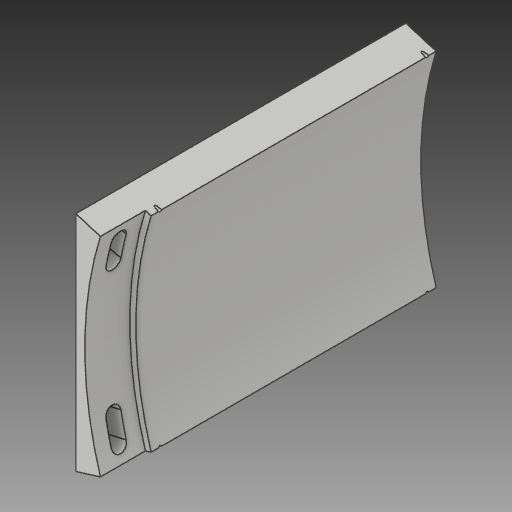
# Autodesk Inventor part: accesorios separador 1
Saved by Autodesk Inventor 2019 (Build 230136000, 136)
## iProperties
Created: 2020-06-11
Part Number: accesorios separador 1
Material: Generic
Document SubType Name: Modeling
Designer: Hugo Albarracin
Density: 1 g/cm^3
Appearance: Default
Author: Hugo Albarracin
Autodesk Inventor part; units mm, degrees
ref_plane "YZ Plane" through (0, 0, 0) normal (1, 0, 0) x (0, 1, 0)
sketch "Sketch1" plane through (0, 0, 0) normal (0, 0, 1) x (1, 0, 0)
  arc A0 (-113.5134, 34.7045) -> (-113.5134, -34.7045) centre (0, 0) ccw
  line L0 (0, 0) -> (-118.7, 0) construction
  line L1 (0, 0) -> (-113.5134, -34.7045) construction
  line L2 (-113.5134, -34.7045) -> (-113.5134, 0) construction
  line L3 (-113.5134, 0) -> (-113.5134, 34.7045) construction
  arc A1 (-116.3823, 35.5816) -> (-116.3823, -35.5816) centre (0, 0) ccw construction
  line L4 (-113.5134, 34.7045) -> (0, 0) construction
  line L5 (-113.5134, -34.7045) -> (-121.7, -37.2074)
  arc A2 (-113.5134, -34.7045) -> (-113.5134, 34.7045) centre (0, 0) ccw construction
  arc A3 (-116.3823, -35.5816) -> (-116.3823, 35.5816) centre (0, 0) ccw construction
  line L6 (-118.7, 0) -> (-121.7, 0) construction
  line L7 (-121.7, 37.2074) -> (-113.5134, 34.7045)
  line L8 (-121.7, 0) -> (-121.7, 37.2074)
  line L9 (-121.7, 0) -> (-121.7, -37.2074)
  dimension "d0" = 237.4
  dimension "d22" = 17
  dimension "d36" = 3
  constraints: 20 end point, 10 point on circle, 4 centre point, 4 vertical, 3 point on line, 2 coincident, 2 collinear, 1 horizontal, 1 tangent
  measures "d0" diameter of A0
  measures "d22" angle of L4 L0
  measures "d36" radial gap between concentric circles of A3 A2
extrude "Extrusion1" add sketch "Sketch1" along normal mid plane 15
sketch "Sketch11" plane through (0, 0, 0) normal (0, 0, 1) x (1, 0, 0)
  line L0 (-121.7, 37.2074) -> (-121.7, -37.2074) projected
  line L1 (0, 0) -> (-115.8526, 25.8431) construction
  line L2 (0, 0) -> (-121.7, 0) construction
  line L3 (0, 0) -> (-115.8526, -25.8431) construction
  circle A0 centre (0, 0) radius 124.6911 construction
  arc A1 (-113.5134, 34.7045) -> (-113.5134, -34.7045) centre (0, 0) ccw projected
  line L4 (-115.8526, 25.8431) -> (-121.7, 27.1474) construction
  line L5 (-115.8526, -25.8431) -> (-121.7, -27.1474) construction
  dimension "d48" = 12.575
  dimension "d49" = 12.575
  constraints: 10 end point, 2 collinear, 2 point on circle, 2 point on line, 1 coincident, 1 midpoint, 3 other
  measures "d48" angle of L2 L1
  measures "d49" angle of L3 L2
ref_plane "Work Plane7" through (-115.8526, 25.8431, 0) normal (0.976, -0.2177, 0) x (0.2177, 0.976, 0)
ref_plane "Work Plane8" through (-115.8526, -25.8431, 0) normal (0.976, 0.2177, 0) x (-0.2177, 0.976, 0)
sketch "Sketch12" plane through (-115.8526, 25.8431, 0) normal (0.976, -0.2177, 0) x (0.2177, 0.976, 0)
  line L0 (-4, 0) -> (4, 0) construction
  line L1 (-4, 2.5) -> (4, 2.5)
  line L2 (4, -2.5) -> (-4, -2.5)
  arc A0 (-4, 2.5) -> (-4, -2.5) centre (-4, 0) ccw
  arc A1 (4, -2.5) -> (4, 2.5) centre (4, 0) ccw
  point P0 (0, 0)
  dimension "d50" = 4
  dimension "d51" = 5
  constraints: 8 end point, 4 point on circle, 4 tangent, 2 centre point, 1 horizontal, 1 midpoint, 1 parallel
  measures "d50" distance of L0.end point (0, 0)
  measures "d51" distance between parallel lines of L1 L2
extrude "Extrusion10" cut sketch "Sketch12" along normal through all both and the other way through all
sketch "Sketch13" plane through (-115.8526, -25.8431, 0) normal (0.976, 0.2177, 0) x (-0.2177, 0.976, 0)
  line L0 (-4, 0) -> (4, 0) construction
  line L1 (-4, 2.5) -> (4, 2.5)
  line L2 (4, -2.5) -> (-4, -2.5)
  arc A0 (-4, 2.5) -> (-4, -2.5) centre (-4, 0) ccw
  arc A1 (4, -2.5) -> (4, 2.5) centre (4, 0) ccw
  point P0 (0, 0)
  dimension "d54" = 5
  dimension "d55" = 4
  constraints: 8 end point, 4 point on circle, 4 tangent, 2 centre point, 1 horizontal, 1 midpoint, 1 parallel
  measures "d54" distance between parallel lines of L2 L1
  measures "d55" distance of L0.start point (0, 0)
extrude "Extrusion11" cut sketch "Sketch13" along normal through all both and the other way through all
ref_plane "Work Plane10" through (-125.6127, 28.0202, 0) normal (0.976, -0.2177, 0) x (0.2177, 0.976, 0)
ref_plane "Work Plane11" through (-125.6127, -28.0202, 0) normal (0.976, 0.2177, 0) x (-0.2177, 0.976, 0)
sketch "Sketch15" plane through (-125.6127, 28.0202, 0) normal (0.976, -0.2177, 0) x (0.2177, 0.976, 0)
  line L0 (5, 0) -> (-5, 0) construction
  line L1 (5, -3.5) -> (-5, -3.5)
  line L2 (-5, 3.5) -> (5, 3.5)
  arc A0 (5, -3.5) -> (5, 3.5) centre (5, 0) ccw
  arc A1 (-5, 3.5) -> (-5, -3.5) centre (-5, 0) ccw
  point P0 (0, 0)
  dimension "d61" = 7
  dimension "d62" = 5
  constraints: 8 end point, 4 point on circle, 4 tangent, 2 centre point, 1 horizontal, 1 midpoint, 1 parallel
  measures "d61" distance between parallel lines of L1 L2
  measures "d62" distance of L0.end point (0, 0)
extrude "Extrusion12" [suppressed]
sketch "Sketch16" plane through (-125.6127, -28.0202, 0) normal (0.976, 0.2177, 0) x (-0.2177, 0.976, 0)
  line L0 (5, 0) -> (-5, 0) construction
  line L1 (5, -3.5) -> (-5, -3.5)
  line L2 (-5, 3.5) -> (5, 3.5)
  arc A0 (5, -3.5) -> (5, 3.5) centre (5, 0) ccw
  arc A1 (-5, 3.5) -> (-5, -3.5) centre (-5, 0) ccw
  point P0 (0, 0)
  dimension "d65" = 7
  dimension "d66" = 5
  constraints: 8 end point, 4 point on circle, 4 tangent, 2 centre point, 1 horizontal, 1 midpoint, 1 parallel
  measures "d65" distance between parallel lines of L1 L2
  measures "d66" distance of L0.end point (0, 0)
extrude "Extrusion13" [suppressed]
sketch "Sketch19" plane through (0, 0, -7.5) normal (0, 0, -1) x (-1, 0, 0)
  arc A0 (113.5134, -34.7045) -> (113.5134, 34.7045) centre (0, 0) ccw projected
  arc A1 (111.6008, -34.1198) -> (111.6008, 34.1198) centre (0, 0) ccw
  line L0 (121.7, 37.2074) -> (121.7, -37.2074) projected
  line L1 (121.7, -37.2074) -> (121.7, 37.2074)
  line L2 (121.7, 37.2074) -> (111.6008, 34.1198)
  line L3 (121.7, -37.2074) -> (111.6008, -34.1198)
  point P0 (0, 0)
  dimension "d75" = 2
  constraints: 6 end point, 2 point on circle, 1 centre point, 1 collinear
  measures "d75" radial gap between concentric circles of A0 A1
extrude "Extrusion15" add sketch "Sketch19" along normal blind 95
sketch "Sketch20" plane through (-121.7, -37.2074, 7.5) normal (-1, 0, 0) x (0, 0, 1)
  line L0 (-107, 3) -> (-18, 3) construction
  line L1 (-18, 3) -> (-18, 71.4148) construction
  line L2 (-18, 71.4148) -> (-107, 71.4148) construction
  line L3 (-107, 71.4148) -> (-107, 3) construction
  line L4 (-15, 2.5029) -> (-15, 71.9119) construction
  line L5 (-110, 74.4148) -> (0, 74.4148) projected
  line L6 (-110, 0) -> (0, 0) projected
  line L7 (-110, 0) -> (-110, 74.4148) projected
  point P0 (-7.5, 37.2074)
  dimension "d78" = 3
  dimension "d79" = 3
  dimension "d80" = 3
  dimension "d81" = 3
  dimension "d82" = 89
  dimension "d83" = 68.4149
  constraints: 8 end point, 2 parallel, 1 horizontal, 1 perpendicular
  measures "d78" distance between parallel lines of L5 L2
  measures "d79" distance between parallel lines of L6 L0
  measures "d80" distance between parallel lines of L7 L3
  measures "d81" distance between parallel lines of L4 L1
  measures "d82" distance of L0.start L0.end
  measures "d83" distance of L2.end L0.start
hole "Hole1" at (-121.7, 34.2074, -99.5) at (-121.7, 34.2074, -10.5) at (-121.7, -34.2074, -99.5) at (-121.7, -34.2074, -10.5) direction (1, 0, 0) diameter 1 depth 25 tip angle 118
equation "\"d49\" = d48"
equation "\"angulo_alabe\" = 130deg"
equation "\"diametro_tubo\" = 232"
equation "\"desfase_a_pin_superior\" = 12"
equation "\"desfase_b_pin_inferior\" = 8"
equation "\"desfase_b_pin_superior\" = 0"
equation "\"diametro_max_soporte\" = 248"
body "Solid1"
